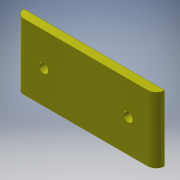
# Autodesk Inventor part: Spessore plastica
Saved by Autodesk Inventor 2018 (Build 220112000, 112)
## iProperties
Created: 2020-05-28
Part Number: Spessore plastica
Material: Generico
Document SubType Name: Modeling
Designer: Francesco
Density: 1 g/cm^3
Appearance: Giallo
Author: Francesco
Autodesk Inventor part; units mm, degrees
ref_plane "YZ Plane" through (0, 0, 0) normal (1, 0, 0) x (0, 1, 0)
ref_plane "XZ Plane" through (0, 0, 0) normal (0, 1, 0) x (-1, 0, 0)
ref_plane "XY Plane" through (0, 0, 0) normal (0, 0, 1) x (1, 0, 0)
sketch "Schizzo1" plane through (0, 0, 0) normal (0, 0, 1) x (1, 0, 0)
  line L0 (-75, 4.5) -> (75, 4.5)
  line L1 (75, 4.5) -> (75, -4.5)
  line L2 (75, -4.5) -> (-75, -4.5)
  line L3 (-75, -4.5) -> (-75, 4.5)
  line L4 (-75, 4.5) -> (75, -4.5) construction
  line L5 (75, 4.5) -> (-75, -4.5) construction
  arc A0 (-75, 4.5) -> (-66, -4.5) centre (-66, 4.5) ccw
  arc A1 (66, -4.5) -> (75, 4.5) centre (66, 4.5) ccw
  point P0 (0, 0)
  dimension "d0" = 150
  dimension "d1" = 9
  dimension "d3" = 9
  dimension "d4" = 9
  constraints: 12 end point, 4 point on circle, 4 point on line, 2 centre point, 2 coincident, 2 midpoint, 2 parallel, 1 horizontal, 1 perpendicular
  measures "d0" distance of L1.end L2.end
  measures "d1" distance of L0.end L1.end
  measures "d3" distance from line of L1 point (66, 4.5)
  measures "d4" distance from line of L3 point (-66, 4.5)
extrude "Estrusione1" add sketch "Schizzo1" along normal blind 70 contours L0 A1 L2 A0
sketch "Schizzo2" plane through (-66, -4.5, 0) normal (0, -1, 0) x (1, 0, 0)
  line L0 (141, 0) -> (141, 70) projected
  line L1 (-9, 0) -> (-9, 70) projected
  point P0 (66, 0)
  point P1 (21, 35)
  point P2 (111, 35)
  point P3 (141, 35)
  dimension "d7" = 30
  dimension "d8" = 30
  dimension "d16" = 90
  constraints: 2 horizontal alignment, 1 midpoint
  measures "d7" distance of point (141, 35) point (111, 35)
  measures "d8" distance from line of L1 point (21, 35)
  measures "d16" distance of point (111, 35) point (21, 35)
hole "Foro1" at (-45, -4.5, 35) at (45, -4.5, 35) direction (0, 1, 0) diameter 10 end through all
